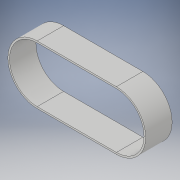
# Autodesk Inventor part: pasek
Saved by Autodesk Inventor 2019 (Build 230136000, 136)
## iProperties
Created: 2020-05-17
Part Number: pasek
Material: Generic
Document SubType Name: Modeling
Designer: estee
Density: 1 g/cm^3
Appearance: Default
Author: estee
Autodesk Inventor part; units mm, degrees
ref_plane "YZ Plane" through (0, 0, 0) normal (1, 0, 0) x (0, 1, 0)
ref_plane "XZ Plane" through (0, 0, 0) normal (0, 1, 0) x (-1, 0, 0)
ref_plane "XY Plane" through (0, 0, 0) normal (0, 0, 1) x (1, 0, 0)
sketch "Sketch1" plane through (0, 0, 0) normal (0, 0, 1) x (1, 0, 0)
  arc A0 (0, 6.274) -> (0, -6.274) centre (0, 0) ccw
  arc A1 (18, -6.274) -> (18, 6.274) centre (18, 0) ccw
  line L0 (0, 6.274) -> (18, 6.274)
  line L1 (0, -6.274) -> (18, -6.274)
  line L2 (18, 6.65) -> (0, 6.65)
  arc A2 (0, 6.65) -> (0, -6.65) centre (0, 0) ccw
  line L3 (0, -6.65) -> (18, -6.65)
  arc A3 (18, -6.65) -> (18, 6.65) centre (18, 0) ccw
  dimension "d0" = 12.548
  dimension "d1" = 12.548
  dimension "d2" = 18
  dimension "d3" = 0.376
  constraints: 8 end point, 8 point on circle, 4 centre point, 2 parallel, 1 coincident, 1 tangent, 3 other
  measures "d0" diameter of A0
  measures "d1" diameter of A1
  measures "d2" distance of A1.centre point (0, 0)
  measures "d3" distance between parallel lines of L0 L2
extrude "Extrusion1" add sketch "Sketch1" along normal blind 6
body "Solid1"
